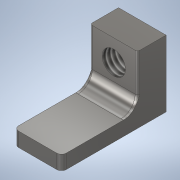
# Autodesk Inventor part: Chip Kick Vorne
Saved by Autodesk Inventor 2020 (Build 240168000, 168)
## iProperties
Part Number: Chip Kick Vorne
Material: Steel, Carbon
Document SubType Name: Modeling
Designer: rYan
Mass: 3.88076 g
Surface Area: 10.5445 cm^2
Volume: 1.43732 cm^3
Density: 7.85 g/cm^3
Appearance: Semi-Polished
Author: rYan
Autodesk Inventor part; units mm, degrees
ref_plane "YZ Plane" through (0, 0, 0) normal (1, 0, 0) x (0, 1, 0)
ref_plane "XZ Plane" through (0, 0, 0) normal (0, 1, 0) x (-1, 0, 0)
ref_plane "XY Plane" through (0, 0, 0) normal (0, 0, 1) x (1, 0, 0)
sketch "Skizze1" plane through (0, 0, 0) normal (1, 0, 0) x (0, 1, 0)
  line L0 (0, 14) -> (-6, 14)
  line L1 (-6, 14) -> (-6, 3)
  line L2 (-22, 0) -> (0, 0)
  line L3 (0, 0) -> (0, 14)
  line L4 (-22, 0) -> (-22, 3)
  line L5 (-22, 3) -> (-6, 3)
  dimension "d0" = 14
  dimension "d1" = 6
  dimension "d2" = 3
  dimension "d3" = 22
  constraints: 12 end point, 2 horizontal, 2 parallel, 1 coincident, 1 perpendicular, 1 vertical
  measures "d0" distance of L2.end L0.start
  measures "d1" distance of L0.start L0.end
  measures "d2" distance of L2.start L4.end
  measures "d3" distance of L2.start L2.end
extrude "Extrusion1" add sketch "Skizze1" along normal mid plane 10
sketch "Skizze2" plane through (-5, 0, 14) normal (0, 1, 0) x (1, 0, 0)
  line L0 (10, 14) -> (10, 0) projected
  line L1 (0, 14) -> (10, 14) projected
  line L2 (0, 0) -> (0, 14) projected
  line L3 (0, 0) -> (10, 0) construction
  line L4 (5, 0) -> (5, 14) construction
  line L5 (10, 0) -> (0, 0) projected
  point P0 (5, 4.5)
  constraints: 2 end point, 1 midpoint, 1 point on line, 1 vertical
hole "Bohrung1" at (0, 0, 9.5) direction (0, -1, 0) diameter 4.917 end through all thread size "M6x1" class "6H" standard "ANSI Metric M Profile"
chamfer "Fase1" [suppressed]
fillet "Rundung1" radius 0.5 2 edges at (5, -6, 8.5) (-5, -6, 8.5)
fillet "Rundung2" radius 1 2 edges at (5, -22, 1.5) (-5, -22, 1.5)
sketch "Skizze5" plane through (-5, 0, 14) normal (0, 1, 0) x (1, 0, 0)
  line L0 (1, 14) -> (1, 11) projected
  line L1 (9, 11) -> (9, 14) projected
  line L2 (0, 14) -> (10, 14) projected
  line L3 (0, 0) -> (0, 14) projected
  line L4 (10, 14) -> (0, 14)
  line L5 (0, 14) -> (0, 11)
  line L6 (0, 11) -> (10, 11)
  line L7 (10, 11) -> (10, 14)
  line L8 (1, 14) -> (9, 14) projected
  line L9 (1, 11) -> (9, 11) projected
  point P0 (5, 14)
  constraints: 8 end point, 2 parallel, 1 horizontal, 1 perpendicular, 1 point on line
fillet "Fillet3" radius 3 2 edges at (4.8536, -5.8536, 3) (-4.8536, -5.8536, 3)
